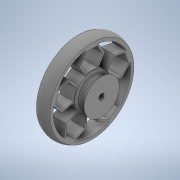
# Autodesk Inventor part: PulleyedWheelV1
Saved by Autodesk Inventor 2020 (Build 240168000, 168)
## iProperties
Created: 2023-12-21
Part Number: PulleyedWheelV1
Material: H TPU
Document SubType Name: Modeling
Designer: smz3rm
Density: 0.941117 g/cm^3
Appearance: Generic(1)
Mass: 5.34144 g
Surface Area: 55.7894 cm^2
Volume: 5.67565 cm^3
d0: 3.000 mm
d1: 1.000 mm
d3: 43.000 mm
d4: 3.000 mm
d6: 18.000 mm
d7: 5.000 mm
d8: 0.00 deg
d9: 43.000 mm
d10: 1.600 mm
d11: 0.800 mm
d16: 7.000 mm
d17: 0.00 deg
d20: 2.500 mm
d24: 1.000 mm
d26: 45.00 deg
Roundedness: 1.000 mm
BaseThickness: 3.000 mm
TopThickness: 1.778 mm
SideThickness: 4.000 mm
BodyWidth: 130.000 mm
BodyLength: 150.000 mm
BodyHeight: 30.000 mm
DriveMotorHeight: 15.000 mm
WheelDia: 45.000 mm
WheelWidth: 7.000 mm
WheelGrooveWidth: 5.000 mm
WheelGrooveDia: 18.000 mm
WheelSlotWidth: 20.000 mm
WheelPulleyDia: 2.500 mm
WheeGuardlSlotWidth: 15.000 mm
Author: smz3rm
Autodesk Inventor part; units mm, degrees
ref_plane "YZ Plane" through (0, 0, 0) normal (1, 0, 0) x (0, 1, 0)
ref_plane "XZ Plane" through (0, 0, 0) normal (0, 1, 0) x (-1, 0, 0)
ref_plane "XY Plane" through (0, 0, 0) normal (0, 0, 1) x (1, 0, 0)
sketch "Sketch1" plane through (0, 0, 0) normal (1, 0, 0) x (0, 1, 0)
  circle A0 centre (0, 0) radius 1.5
  line L0 (-30.1, 0) -> (30.1, 0) projected
  line L1 (1.118, -1) -> (-1.118, -1)
  circle A1 centre (0, 0) radius 9
  circle A2 centre (0, 0) radius 21.5
  circle A3 centre (0, 0) radius 18.5
  dimension "d0" = 3
  dimension "d1" = 1
  dimension "d3" = 43
  dimension "d4" = 3
  dimension "d6" = 18
  constraints: 4 centre point, 4 coincident, 2 end point, 2 point on circle, 1 horizontal
  measures "d0" diameter of A0
  measures "d1" distance between parallel lines of L0 L1
  measures "d3" diameter of A2
  measures "d4" radial gap between concentric circles of A2 A3
  measures "d6" diameter of A1
extrude "Extrusion1" add sketch "Sketch1" along normal blind 5 contours L1 A0 | A0 L0 A1 | L0 A1 A0
sketch "Sketch3" plane through (0, 0, 0) normal (0, 0, 1) x (1, 0, 0)
  line L0 (0, 9) -> (5, 9) projected
  line L1 (-0.9, 0) -> (5.4, 0) projected
  circle A0 centre (1.7822, 7.75) radius 1.25
  line L2 (0.5662, 7.4607) -> (0.2, 9)
  line L3 (0, 9) -> (5, 9) projected
  line L4 (0, 10) -> (5, 10) projected
  line L5 (0, 9) -> (5, 9) projected
  line L6 (4.8, 9) -> (2.6661, 6.8661)
  line L7 (4.8, 9) -> (4.8, 9)
  line L8 (4.8, 9) -> (5, 9)
  line L9 (5, -9) -> (5, 9) projected
  line L10 (5, 9) -> (5, 9)
  line L11 (0, -9) -> (0, 9) projected
  line L12 (0.2, 9) -> (0, 9)
  point P0 (0, 0)
  point P1 (1.7822, 9)
  point P2 (4.8, 9)
  dimension "d20" = 2.5
  dimension "d26" = 45
  dimension "d28" = 0.2
  constraints: 12 end point, 3 perpendicular, 3 tangent, 2 collinear, 2 point on circle, 2 point on line, 1 centre point, 1 vertical, 3 other
  measures "d20" diameter of A0
  measures "d26" angle of L0 L6
  measures "d28" distance of L0.end L6.start
revolve "Revolution1" cut sketch "Sketch3" angle 360 about axis through (-10, 0, 0) along (-1, 0, 0) contours L0 A0 L2 | L0 L6 A0 | A0
sketch "Sketch2" plane through (0, 0, 0) normal (-1, 0, 0) x (0, 0, 1)
  circle A0 centre (0, 0) radius 21.5
  circle A1 centre (0, 0) radius 19.9
  circle A2 centre (0, 0) radius 9 projected
  line L0 (-1, 1.118) -> (-1, -1.118) projected
  arc A3 (-1, -1.118) -> (-1, 1.118) centre (0, 0) ccw projected
  line L1 (3.2444, 19.6337) -> (6.4888, 14.0143)
  line L2 (6.4888, 14.0143) -> (3.2444, 8.3949)
  line L3 (3.2444, 8.3949) -> (-3.2444, 8.3949)
  line L4 (-3.2444, 8.3949) -> (-6.4888, 14.0143)
  line L5 (-6.4888, 14.0143) -> (-3.2444, 19.6337)
  line L6 (-3.2444, 19.6337) -> (3.2444, 19.6337)
  line L7 (0, -30.1) -> (0, 30.1) projected
  line L8 (-2.7825, 18.8337) -> (-5.565, 14.0143)
  line L9 (-5.565, 14.0143) -> (-2.7825, 9.1949)
  line L10 (-2.7825, 9.1949) -> (2.7825, 9.1949)
  line L11 (2.7825, 9.1949) -> (5.565, 14.0143)
  line L12 (5.565, 14.0143) -> (2.7825, 18.8337)
  line L13 (2.7825, 18.8337) -> (-2.7825, 18.8337)
  line L14 (-17.6702, 9.1528) -> (-11.3233, 10.5018)
  line L15 (-19.6754, 2.9816) -> (-17.6702, 9.1528)
  line L16 (-15.3335, -1.8405) -> (-19.6754, 2.9816)
  line L17 (-8.9866, -0.4914) -> (-15.3335, -1.8405)
  line L18 (-15.0481, -0.962) -> (-9.6047, 0.1951)
  line L19 (-9.6047, 0.1951) -> (-7.885, 5.4877)
  line L20 (-7.885, 5.4877) -> (-11.6087, 9.6233)
  line L21 (-11.3233, 10.5018) -> (-6.9814, 5.6798)
  line L22 (-6.9814, 5.6798) -> (-8.9866, -0.4914)
  line L23 (-11.6087, 9.6233) -> (-17.0521, 8.4663)
  line L24 (-17.0521, 8.4663) -> (-18.7718, 3.1736)
  line L25 (-18.7718, 3.1736) -> (-15.0481, -0.962)
  line L26 (-14.1652, -13.977) -> (-13.4869, -7.5238)
  line L27 (-8.9157, -17.791) -> (-14.1652, -13.977)
  line L28 (-2.9879, -15.1518) -> (-8.9157, -17.791)
  line L29 (-2.3096, -8.6986) -> (-2.9879, -15.1518)
  line L30 (-3.7352, -14.6088) -> (-3.1535, -9.0743)
  line L31 (-3.1535, -9.0743) -> (-7.6557, -5.8033)
  line L32 (-7.6557, -5.8033) -> (-12.7396, -8.0668)
  line L33 (-13.4869, -7.5238) -> (-7.5591, -4.8846)
  line L34 (-7.5591, -4.8846) -> (-2.3096, -8.6986)
  line L35 (-12.7396, -8.0668) -> (-13.3213, -13.6013)
  line L36 (-13.3213, -13.6013) -> (-8.8191, -16.8723)
  line L37 (-8.8191, -16.8723) -> (-3.7352, -14.6088)
  line L38 (8.9157, -17.791) -> (2.9879, -15.1518)
  line L39 (14.1652, -13.977) -> (8.9157, -17.791)
  line L40 (13.4869, -7.5238) -> (14.1652, -13.977)
  line L41 (7.5591, -4.8846) -> (13.4869, -7.5238)
  line L42 (12.7396, -8.0668) -> (7.6557, -5.8033)
  line L43 (7.6557, -5.8033) -> (3.1535, -9.0743)
  line L44 (3.1535, -9.0743) -> (3.7352, -14.6088)
  line L45 (2.9879, -15.1518) -> (2.3096, -8.6986)
  line L46 (2.3096, -8.6986) -> (7.5591, -4.8846)
  line L47 (3.7352, -14.6088) -> (8.8191, -16.8723)
  line L48 (8.8191, -16.8723) -> (13.3213, -13.6013)
  line L49 (13.3213, -13.6013) -> (12.7396, -8.0668)
  line L50 (19.6754, 2.9816) -> (15.3335, -1.8405)
  line L51 (17.6702, 9.1528) -> (19.6754, 2.9816)
  line L52 (11.3233, 10.5018) -> (17.6702, 9.1528)
  line L53 (6.9814, 5.6798) -> (11.3233, 10.5018)
  line L54 (11.6087, 9.6233) -> (7.885, 5.4877)
  line L55 (7.885, 5.4877) -> (9.6047, 0.1951)
  line L56 (9.6047, 0.1951) -> (15.0481, -0.962)
  line L57 (15.3335, -1.8405) -> (8.9866, -0.4914)
  line L58 (8.9866, -0.4914) -> (6.9814, 5.6798)
  line L59 (15.0481, -0.962) -> (18.7718, 3.1736)
  line L60 (18.7718, 3.1736) -> (17.0521, 8.4663)
  line L61 (17.0521, 8.4663) -> (11.6087, 9.6233)
  point P0 (0, 14.0143)
  point P1 (3.2444, 8.3949)
  point P2 (-17.6702, 9.1528)
  point P3 (-6.9814, 5.6798)
  point P4 (-19.6754, 2.9816)
  point P5 (-8.9866, -0.4914)
  point P6 (-7.5591, -4.8846)
  point P7 (-14.1652, -13.977)
  point P8 (-8.9157, -17.791)
  point P9 (-2.3096, -8.6986)
  point P10 (2.3096, -8.6986)
  point P11 (8.9157, -17.791)
  point P12 (14.1652, -13.977)
  point P13 (7.5591, -4.8846)
  point P14 (8.9866, -0.4914)
  point P15 (19.6754, 2.9816)
  point P16 (17.6702, 9.1528)
  point P17 (6.9814, 5.6798)
  dimension "d9" = 43
  dimension "d10" = 1.6
  dimension "d11" = 0.8
  dimension "d31" = 360
  constraints: 120 end point, 2 centre point, 2 coincident, 2 point on circle, 1 point on line, 141 other
  measures "d9" diameter of A0
  measures "d10" radial gap between concentric circles of A0 A1
  measures "d11" distance between parallel lines of L5 L8
extrude "Extrusion2" add sketch "Sketch2" along normal blind 7 contours A0 L7 A1 | L7 A1 A0 | L7 L6 A1 | A1 L6 L7 | L1 L2 A2 L7 L10 L11 L12 L13 L6 | L6 L7 L13 L8 L9 L10 A2 L4 L5 | A1 L27 | L27 L26 L33 A2 L29 L28 | L39 A1 | L38 L45 A2 L41 L40 L39 | L7 A3 L3 A2 L58 L46 | A2 L34 L22 L3 L7 A3 L0 | A1 L51 | L51 L50 L57 A2 L53 L52 | L15 A1 | L14 L21 A2 L17 L16 L15 | A2 L34 | L46 A2 | L3 L7 A2 | A2 L7 L3 | A2 L58 | L22 A2
sketch "Sketch4" plane through (0, 0, 0) normal (0, 0, 1) x (1, 0, 0)
  line L0 (0, 21.5) -> (-7, 21.5) projected
  line L1 (-7, 21.5) -> (-7, -21.5) projected
  arc A0 (0, 21.5) -> (-7, 21.5) centre (-3.5, 15.875) ccw
  line L2 (-8.4, 0) -> (1.4, 0) projected
  point P0 (0, 0)
  point P1 (-3.5, 22.5)
  dimension "d24" = 1
  constraints: 3 point on circle, 1 centre point
  measures "d24" distance from line of L0 point (-3.5, 22.5)
revolve "Revolution2" add sketch "Sketch4" angle 360 about axis through (-10, 0, 0) along (1, 0, 0)
equation "\"d6\" = WheelGrooveDia"
equation "\"d7\" = WheelGrooveWidth"
equation "\"d20\" = WheelPulleyDia"
equation "\"d9\" = WheelDia - 2 * Roundedness"
equation "\"d16\" = WheelWidth"
equation "\"d24\" = Roundedness"
equation "\"Roundedness\" = 1"
equation "\"WheelGrooveDia\" = 18"
equation "\"WheelGrooveWidth\" = 5"
equation "\"WheelPulleyDia\" = 2.5"
equation "\"WheelDia\" = 45"
equation "\"WheelWidth\" = 7"
body "Solid1"
